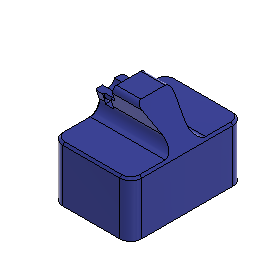
side entry (Autodesk Fusion 360 design; units mm, degrees)
Autodesk Fusion 360 part; units mm, degrees
ref_plane "WorkPlane3" through (0, 0, 20) normal (0, 0, 1) x (1, 0, 0)
sketch "Sketch1" plane through (0, 0, 20) normal (0, 0, 1) x (-1, 0, 0)
  circle A0 centre (13.5, -22) radius 1.4
  circle A1 centre (-13.5, -22) radius 1.4
  circle A2 centre (13.5, 22) radius 1.4
  circle A3 centre (-13.5, 22) radius 1.4
  arc A4 (-14, 25.5) -> (-17, 22.5) centre (-14, 22.5) ccw
  arc A5 (17, 22.5) -> (14, 25.5) centre (14, 22.5) ccw
  arc A6 (14, -25.5) -> (17, -22.5) centre (14, -22.5) ccw
  arc A7 (-17, -22.5) -> (-14, -25.5) centre (-14, -22.5) ccw
  line L0 (14, -25.5) -> (-14, -25.5)
  line L1 (17, -22.5) -> (17, 22.5)
  line L2 (14, 25.5) -> (-14, 25.5)
  line L3 (-17, 22.5) -> (-17, -22.5)
  line L4 (13.5, -22) -> (-13.5, 22) construction
  line L5 (-13.5, -22) -> (13.5, 22) construction
  line L6 (14, -22.5) -> (-14, 22.5) construction
  line L7 (13.5, -22) -> (-13.5, -22) construction
  line L8 (-13.5, -22) -> (-13.5, 22) construction
  line L9 (-13.5, 22) -> (13.5, 22) construction
  line L10 (13.5, 22) -> (13.5, -22) construction
  arc A8 (-19.5, -22.5) -> (-14, -28) centre (-14, -22.5) ccw
  line L11 (14, -28) -> (-14, -28)
  arc A9 (14, -28) -> (19.5, -22.5) centre (14, -22.5) ccw
  line L12 (19.5, -22.5) -> (19.5, 22.5)
  arc A10 (19.5, 22.5) -> (14, 28) centre (14, 22.5) ccw
  line L13 (14, 28) -> (-14, 28)
  arc A11 (-14, 28) -> (-19.5, 22.5) centre (-14, 22.5) ccw
  line L14 (-19.5, 22.5) -> (-19.5, -22.5)
  circle A12 centre (-13.5, -22) radius 3.5
  circle A13 centre (13.5, -22) radius 3.5
  circle A14 centre (-13.5, 22) radius 3.5
  circle A15 centre (13.5, 22) radius 3.5
  line L15 (-13.5, 18.5) -> (-17, 18.5)
  line L16 (13.5, 18.5) -> (17, 18.5)
  line L17 (10, 22) -> (10, 25.5)
  line L18 (-10, 22) -> (-10, 25.5)
  line L19 (-10, -22) -> (-10, -25.5)
  line L20 (-13.5, -18.5) -> (-17, -18.5)
  line L21 (10, -22) -> (10, -25.5)
  line L22 (13.5, -18.5) -> (17, -18.5)
  line L23 (10, 23.5) -> (-10, 23.5)
  line L24 (10, -23.5) -> (-10, -23.5)
  dimension "d219" = 27
  dimension "d220" = 44
  dimension "d221" = 51
  dimension "d222" = 34
  dimension "d223" = 3
  dimension "d224" = -2.5
  dimension "d16" = 2.8
  dimension "d17" = 2
  dimension "d18" = 2
  constraint tangent A7 L0
  constraint tangent A5 L1
  constraint tangent A4 L2
  constraint tangent A7 L3
  constraint coincident A0.centre L4.start
  constraint coincident A3.centre L4.end
  constraint coincident A1.centre L5.start
  constraint coincident A2.centre L5.end
  constraint equal A6 A7
  constraint equal A4 A6
  constraint equal A5 A6
  constraint coincident A6.centre L6.start
  constraint coincident A4.centre L6.end
  constraint midpoint L5 L6
  constraint vertical L3
  constraint horizontal L0
  constraint tangent A6 L0
  constraint tangent A6 L1
  constraint tangent A5 L2
  constraint tangent A4 L3
  constraint horizontal L7
  constraint vertical L8
  constraint horizontal L9
  constraint vertical L10
  constraint coincident A1.centre L8
  constraint midpoint origin L5
  constraint equal A0 A1
  constraint equal A1 A2
  constraint equal A1 A3
  constraint concentric A1 A12
  constraint tangent L3 A12
  constraint concentric A0 A13
  constraint tangent L1 A13
  constraint concentric A3 A14
  constraint concentric A2 A15
  constraint tangent L3 A14
  constraint tangent L1 A15
  constraint coincident A14 L15.start
  constraint coincident L8 L15.start
  constraint coincident L3 L15.end
  constraint tangent A14 L15
  constraint coincident L10 L16.start
  constraint coincident A15 L16.start
  constraint coincident L1 L16.end
  constraint tangent A15 L16
  constraint coincident A15 L17.start
  constraint coincident L9 L17.start
  constraint coincident L2 L17.end
  constraint tangent A15 L17
  constraint coincident L9 L18.start
  constraint coincident A14 L18.start
  constraint coincident L2 L18.end
  constraint tangent A14 L18
  constraint coincident A12 L19.start
  constraint coincident L7 L19.start
  constraint coincident L0 L19.end
  constraint coincident L8 L20.start
  constraint coincident A12 L20.start
  constraint coincident L3 L20.end
  constraint tangent A12 L20
  constraint tangent A12 L19
  constraint coincident A13 L21.start
  constraint coincident L7 L21.start
  constraint coincident L0 L21.end
  constraint tangent A13 L21
  constraint coincident A13 L22.start
  constraint coincident L10 L22.start
  constraint coincident L1 L22.end
  constraint tangent A13 L22
  constraint coincident L17 L23.start
  constraint coincident L18 L23.end
  constraint perpendicular L18 L23
  constraint coincident L21 L24.start
  constraint coincident L19 L24.end
  constraint perpendicular L19 L24
  measures "d219" distance of A0.centre A1.centre
  measures "d220" distance of A0.centre A2.centre
  measures "d221" distance of L0 L2
  measures "d222" distance of L1 L3
  measures "d223" radius of A6
  measures "d16" diameter of A1
  measures "d17" distance of L2 L23
  measures "d18" distance of L0 L24
extrude "Extrude3" add sketch "Sketch1" along normal blind 24 contours A4 L2 L3 A14 | L2 A14 L18 | A14 | L3 A14 L15 | L2 L17 L18 L23 | L2 A15 L17 | L3 A12 L20 | A5 L1 L2 A15 | A15 | A7 L0 L3 A12 | A12 | L1 A15 L16 | L0 A12 L19 | L0 L19 L21 L24 | L1 A13 L22 | L0 A13 L21 | A13 | A6 L0 L1 A13 | A8 L11 A9 L12 A10 L13 A11 L14
sketch "Sketch2" plane through (0, 0, 44) normal (0, 0, 1) x (-1, 0, 0)
  line L0 (-17, -18.5) -> (-17, 18.5)
  line L1 (17, 18.5) -> (17, -18.5)
  arc A0 (14, -28) -> (19.5, -22.5) centre (14, -22.5) ccw
  line L2 (19.5, -22.5) -> (19.5, 22.5)
  arc A1 (19.5, 22.5) -> (14, 28) centre (14, 22.5) ccw
  line L3 (14, 28) -> (-14, 28)
  arc A2 (-14, 28) -> (-19.5, 22.5) centre (-14, 22.5) ccw
  line L4 (-19.5, 22.5) -> (-19.5, -22.5)
  arc A3 (-19.5, -22.5) -> (-14, -28) centre (-14, -22.5) ccw
  line L5 (-14, -28) -> (14, -28)
  circle A4 centre (-13.5, 22) radius 1.4
  circle A5 centre (-13.5, -22) radius 1.4
  circle A6 centre (13.5, -22) radius 1.4
  circle A7 centre (13.5, 22) radius 1.4
  arc A8 (13.5, -18.5) -> (10, -22) centre (13.5, -22) ccw
  line L6 (10, -22) -> (10, -23.5)
  line L7 (-10, -23.5) -> (-10, -22)
  arc A9 (-10, -22) -> (-13.5, -18.5) centre (-13.5, -22) ccw
  line L8 (-13.5, -18.5) -> (-17, -18.5)
  line L9 (-17, 18.5) -> (-13.5, 18.5)
  arc A10 (-13.5, 18.5) -> (-10, 22) centre (-13.5, 22) ccw
  line L10 (-10, 22) -> (-10, 23.5)
  line L11 (10, 23.5) -> (10, 22)
  arc A11 (10, 22) -> (13.5, 18.5) centre (13.5, 22) ccw
  line L12 (13.5, 18.5) -> (17, 18.5)
  line L13 (17, -18.5) -> (13.5, -18.5)
  line L14 (10, -23.5) -> (-10, -23.5)
  line L15 (-10, 23.5) -> (10, 23.5)
extrude "Extrude5" add sketch "Sketch2" along normal blind 3 contours L0 L1 A8 L6 L7 A9 L8 L9 A10 L10 L11 A11 L12 L13 L14 L15 | A0 L2 A1 L3 A2 L4 A3 L5 | A4 | A5 | A6 | A7
ref_plane "WorkPlane4" through (0, 0, 33.5) normal (-1, 0, 0) x (0, -1, 0)
sketch "Sketch3" plane through (0, 0, 0) normal (-1, 0, 0) x (0, 1, 0)
  circle A0 centre (10, -51.5) radius 4.5
  line L0 (-10, -51.5) -> (-10, -47) construction
  line L1 (10, -51.5) -> (10, -47) construction
  circle A1 centre (-10, -51.5) radius 4.5
  circle A2 centre (6, -61) radius 2
  circle A3 centre (-6, -61) radius 2
  line L2 (6, -61) -> (-6, -61) construction
  line L3 (-6, -61) -> (0, -61) construction
  line L4 (0, -47) -> (0, -61) construction
  line L5 (5.68, -52.76) -> (7.92, -60.44)
  line L6 (-5.68, -52.76) -> (-7.92, -60.44)
  line L7 (6, -63) -> (-6, -63)
  line L8 (-10, -47) -> (10, -47) construction
  line L9 (-28, -47) -> (28, -47)
  dimension "d102" = 9
  dimension "d104" = 12
  dimension "d105" = 4
  dimension "d106" = 14
  dimension "d225" = 10
  dimension "d226" = 10
  constraint coincident A0.centre L1.start
  constraint vertical L1
  constraint vertical L0
  constraint coincident L0.start A1.centre
  constraint equal A0 A1
  constraint coincident A2.centre L2.start
  constraint coincident A3.centre L2.end
  constraint horizontal L2
  constraint midpoint L2 L3.end
  constraint vertical L4
  constraint coincident A0 L5.start
  constraint tangent A0 L5
  constraint coincident A2 L5.end
  constraint coincident A1 L6.start
  constraint tangent A1 L6
  constraint coincident A3 L6.end
  constraint tangent A3 L6
  constraint tangent A2 L5
  constraint equal A2 A3
  constraint coincident A2 L7.start
  constraint tangent A2 L7
  constraint coincident A3 L7.end
  constraint tangent A3 L7
  constraint coincident A0 L1.end
  constraint coincident L0.end A1
  constraint tangent A0 L8
  constraint midpoint L4.start L8
  constraint collinear L8 L9
  constraint midpoint L4.start L9
  measures "d102" diameter of A0
  measures "d104" distance of A2.centre A3.centre
  measures "d105" diameter of A2
  measures "d106" distance of L4.start L3.end
  measures "d225" distance of L0.start L4
  measures "d226" distance of L1 L4
extrude "Extrude6" add sketch "Sketch3" along normal blind -19.5 and the other way blind -19.5 contours A0 A1 A2 A3 L5 L6 L7 L9 | A2 | A3
ref_plane "WorkPlane1" through (0, 0, 33.25) normal (0, 1, 0) x (-1, 0, 0)
sketch "Sketch4" plane through (0, 0, 0) normal (0, 1, 0) x (-1, 0, 0)
  arc A0 (11, 57) -> (1, 47) centre (11, 47) ccw
  line L0 (1, 47) -> (1, 38)
  line L1 (11, 57) -> (39.9841, 57)
  point P0 (27.5, 47)
  point P1 (-19, 47)
  dimension "d2" = 9
  dimension "d3" = 10
  dimension "d4" = 20
  constraint vertical L0
  constraint tangent A0 L0
  constraint tangent A0 L1
  constraint horizontal L1
  measures "d2" distance of A0.end L0.end
  measures "d3" radius of A0
  measures "d4" distance of P1 L0
ref_plane "WorkPlane5" through (-39.1567, 0, 57) normal (-1, 0, 0) x (0, 0, -1)
sketch "Sketch5" plane through (-39.1567, 0, 57) normal (-1, 0, 0) x (0, 0, -1)
  circle A0 centre (0, 0) radius 3
  dimension "d111" = 6
  constraint coincident A0.centre origin
  measures "d111" diameter of A0
sweep "Sweep1" cut profiles "Sketch5" path "Sketch4" along L0 A0 L1 section 1
fillet "Fillet5" radius 3 1 edges at (1.797, 1.0848, 44)
sketch "Sketch8" plane through (-19.5, 0, 0) normal (-1, 0, 0) x (0, -1, 0)
  arc A0 (7.92, 60.44) -> (6, 63) centre (6, 61) ccw
  line L0 (5.68, 52.76) -> (7.92, 60.44)
  arc A1 (5.68, 52.76) -> (10, 47) centre (10, 51.5) ccw
  line L1 (-7.92, 60.44) -> (-5.68, 52.76)
  arc A2 (-6, 63) -> (-7.92, 60.44) centre (-6, 61) ccw
  line L2 (6, 63) -> (-6, 63)
  circle A3 centre (0, 57) radius 3
  line L3 (-6.8, 56.6) -> (6.8, 56.6)
  arc A4 (-10, 47) -> (-5.68, 52.76) centre (-10, 51.5) ccw
  line L4 (-22.5, 20) -> (22.5, 20)
  line L5 (22.5, 20) -> (22.5, 47)
  line L6 (22.5, 47) -> (10, 47)
  line L7 (-10, 47) -> (-22.5, 47)
  line L8 (-22.5, 47) -> (-22.5, 20)
  constraint midpoint L1 L3.start
  constraint midpoint L0 L3.end
extrude "Extrude9" cut sketch "Sketch8" against normal blind 10 contours A0 L0 L1 A2 L2 A3 L3
delete_face "DeleteFace1" 1 faces at (-10.5, 0, 60)
sketch "Sketch12" plane through (0, 0, 0) normal (1, 0, 0) x (0, 1, 0)
  line L0 (-28, 47) -> (-4.3657, 70.6343)
  line L1 (-4.3657, 70.6343) -> (-28, 70.6343)
  line L2 (-28, 70.6343) -> (-28, 47)
  line L3 (-28, 47) -> (-28, 20)
  point P0 (27, 47)
  point P1 (-27, 47)
  point P2 (-28, 47)
  dimension "d10" = 45
  dimension "d11" = 23.6343
  constraint coincident P2 L0.start
  constraint perpendicular L1 L2
  constraint vertical L2
  measures "d10" angle of L0 L2
  measures "d11" horizontal distance of L0.end L1.end
sketch "Sketch13" plane through (0, 0, 56.6) normal (0, 0, 1) x (-1, 0, 0)
  spline S0 degree 3 poles (11, 2.9732) (10.5349, 2.9732) (9.9994, 2.9793) (9.5, 2.9866) knots 0 0 0 0 0.139545 0.139545 0.139545 0.139545
  line L0 (11, 2.9732) -> (19.5, 2.9732)
  line L1 (19.5, 2.9732) -> (19.5, 6.8)
  line L2 (19.5, 6.8) -> (9.5, 6.8)
  line L3 (9.5, 6.8) -> (9.5, 2.9866)
  line L4 (15.5, -6.8) -> (11.5, -6.8)
  line L5 (11.5, -6.8) -> (11.5, -5.8)
  line L6 (11.5, -5.8) -> (15.5, -5.8)
  line L7 (15.5, -5.8) -> (15.5, -6.8)
  line L8 (9.5, -2.9866) -> (9.5, -6.8)
  line L9 (19.5, -6.8) -> (9.5, -6.8)
  dimension "d24" = 2
  dimension "d25" = 4
  dimension "d26" = 1
  constraint horizontal L4
  constraint vertical L5
  constraint horizontal L6
  constraint vertical L7
  constraint collinear L4 L9
  measures "d24" distance of L5.end L8
  measures "d25" distance of L4.start L4.end
  measures "d26" distance of L4.start L6.end
extrude "Extrude12" cut sketch "Sketch13" against normal blind 5 contours L4 L5 L6 L7 L9
mirror "Mirror1" about plane through (0, 0, 33.25) normal (0, 1, 0) of "Extrude12"
sketch "Sketch14" plane through (0, 0, 0) normal (0, 1, 0) x (1, 0, 0)
  line L0 (-15.5, -56.6) -> (-11.5, -56.6)
  line L1 (-11.5, -53.6) -> (-15.5, -53.6)
  line L2 (-15.5, -53.6) -> (-15.5, -51.6)
  line L3 (-15.5, -51.6) -> (-11.5, -51.6)
  line L4 (-11.5, -51.6) -> (-11.5, -53.6)
  line L5 (-13.5, -56.6) -> (-13.5, -53.6) construction
  dimension "d31" = 4
  dimension "d32" = 3
  dimension "d33" = 2
  constraint horizontal L1
  constraint vertical L2
  constraint horizontal L3
  constraint vertical L4
  constraint midpoint L0 L5.start
  constraint midpoint L1 L5.end
  constraint vertical L5
  measures "d31" distance of L2.end L3.end
  measures "d32" distance of L0 L1
  measures "d33" distance of L1.start L3.end
extrude "Extrude13" cut sketch "Sketch14" along normal through all and the other way through all
fillet "Fillet8" radius 1 2 edges at (-13.5, -5.8, 53.6) (-13.5, 5.8, 53.6)
sketch "Sketch15" plane through (0, 0, 0) normal (0, 1, 0) x (1, 0, 0)
  line L0 (-9.5, -63) -> (19.5, -63)
  line L1 (19.5, -63) -> (-9.5, -63)
  line L2 (19.5, -20) -> (19.5, -47)
  line L3 (19.5, -47) -> (19.5, -52.76)
  line L4 (19.5, -52.76) -> (19.5, -60.44)
  line L5 (19.5, -63) -> (19.5, -60.44)
  line L6 (19.5, -63) -> (19.5, -60.44)
  line L7 (19.5, -60.44) -> (19.5, -52.76)
  line L8 (19.5, -47) -> (19.5, -52.76)
  line L9 (19.5, -47) -> (19.5, -20)
  line L10 (19.5, -46) -> (2.5, -63)
  point P0 (19.5, -47)
  dimension "d39" = 45
  dimension "d40" = 1
  constraint coincident L9 L10.start
  constraint coincident L1 L10.end
  measures "d39" angle of L1 L10
  measures "d40" distance of P0 L10.start
extrude "Extrude14" cut sketch "Sketch15" against normal through all and the other way through all
chamfer "Chamfer9" distance 1 angle 45 12 edges at (0, -28, 47) (16.5355, -27.3807, 47) (-19.5, -6.24, 54.68) (-19.5, -6.4, 48.8) (-19.5, -16.25, 47) (-17.8891, -26.3891, 47) (0, 28, 47) (-17.8891, 26.3891, 47) (-19.5, 16.25, 47) (-19.5, 6.4, 48.8) (-19.5, 6.24, 54.68) (16.5355, 27.3807, 47)
chamfer "Chamfer8" [suppressed]
named bodies: "Cover 6 way Side entry"
